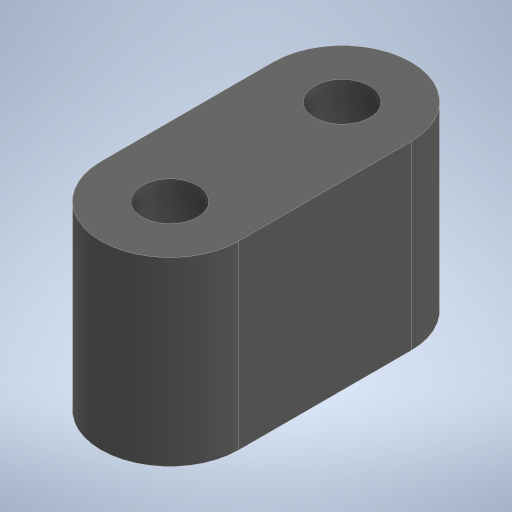
# Autodesk Inventor part: spacer_2_hole
Saved by Autodesk Inventor 2024.1 (Build 281209000, 209)
## iProperties
Created: 2025-10-20
Part Number: spacer_2_hole
Material: 一般
Document SubType Name: Modeling
Designer: hibik
Density: 1 g/cm^3
Appearance: 既定
Author: hibik
Autodesk Inventor part; units mm, degrees
ref_plane "YZ Plane" through (0, 0, 0) normal (1, 0, 0) x (0, 1, 0)
ref_plane "XZ Plane" through (0, 0, 0) normal (0, 1, 0) x (-1, 0, 0)
ref_plane "XY Plane" through (0, 0, 0) normal (0, 0, 1) x (1, 0, 0)
sketch "スケッチ1" plane through (0, 0, 0) normal (0, 1, 0) x (-1, 0, 0)
  circle A0 centre (0, 5) radius 1.6
  circle A1 centre (0, -5) radius 1.6
  line L0 (5.6, 0) -> (-5.6, 0) projected
  line L1 (0, -5) -> (0, 5) construction
  line L2 (4, -5) -> (4, 5)
  line L3 (-4, 5) -> (-4, -5)
  arc A2 (-4, -5) -> (4, -5) centre (0, -5) ccw
  arc A3 (4, 5) -> (-4, 5) centre (0, 5) ccw
  point P0 (0, 0)
  dimension "d0" = 3.2
  dimension "d1" = 3.2
  dimension "d2" = 10
  dimension "d3" = 4
  constraints: 8 end point, 4 centre point, 4 point on circle, 4 tangent, 2 vertical alignment, 1 midpoint, 1 parallel, 1 symmetric about line, 1 vertical
  measures "d0" diameter of A0
  measures "d1" diameter of A1
  measures "d2" distance of A1.centre L1.end
  measures "d3" radius of A3
extrude "押し出し1" add sketch "スケッチ1" along normal blind 10.5
